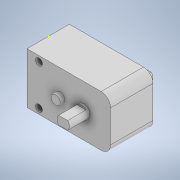
# Autodesk Inventor part: TT motor output
Saved by Autodesk Inventor 2022 (Build 260153070, 153G)
## iProperties
Created: 2021-11-27
Part Number: TT motor output
Material: Generic
Document SubType Name: Modeling
Designer: a laptop
Density: 1 g/cm^3
Appearance: Default
Author: a laptop
Autodesk Inventor part; units mm, degrees
ref_plane "YZ Plane" through (0, 0, 0) normal (1, 0, 0) x (0, 1, 0)
ref_plane "XZ Plane" through (0, 0, 0) normal (0, 1, 0) x (-1, 0, 0)
ref_plane "XY Plane" through (0, 0, 0) normal (0, 0, 1) x (1, 0, 0)
sketch "Sketch1" plane through (0, 0, 0) normal (0, 0, 1) x (1, 0, 0)
  line L0 (0, 0) -> (32.375, 0)
  line L1 (36.5, 0) -> (36.5, -4.125)
  line L2 (36.5, -22.25) -> (0, -22.25)
  line L3 (0, -22.25) -> (0, -11.125)
  line L4 (0, -11.125) -> (36.5, -11.125) construction
  line L5 (0, -11.125) -> (0, 0)
  circle A0 centre (14.5, -11.125) radius 2
  circle A1 centre (5.25, -2.375) radius 1.5
  arc A2 (36.5, -4.125) -> (32.375, 0) centre (32.375, -4.125) ccw
  line L6 (32.375, 0) -> (36.5, 0)
  line L7 (36.5, -4.125) -> (36.5, -22.25)
  arc A3 (32.375, -22.25) -> (36.5, -18.125) centre (32.375, -18.125) ccw
  circle A4 centre (5.25, -19.875) radius 1.5
  circle A5 centre (24.8, -11.125) radius 2.7
  line L8 (22.8334, -9.275) -> (26.7666, -9.275)
  line L9 (26.7666, -12.975) -> (22.8334, -12.975)
  point P0 (36.5, -18.125)
  dimension "d6" = 4
  dimension "d8" = 3
  dimension "d11" = 5.25
  dimension "d12" = 22.25
  dimension "d13" = 8.75
  dimension "d16" = 14.5
  dimension "d17" = 14
  dimension "d18" = 36.5
  dimension "d19" = 3.7
  dimension "d28" = 5.4
  dimension "d29" = 11.7
  constraints: 20 end point, 9 point on circle, 7 parallel, 6 centre point, 6 perpendicular, 6 point on line, 4 symmetric about line, 3 equal length, 3 horizontal, 2 tangent, 1 coincident, 1 horizontal alignment, 1 vertical alignment, 2 other
  measures "d6" diameter of A0
  measures "d8" diameter of A1
  measures "d11" distance from line of L5 A1.centre
  measures "d12" distance of L1.start L2.start
  measures "d13" distance from line of L4 A1.centre
  measures "d16" distance from line of L3 A0.centre
  measures "d17" distance of A3.end A2.start
  measures "d18" distance of L0.start L1.start
  measures "d19" distance between parallel lines of L9 L8
  measures "d28" diameter of A5
  measures "d29" distance from line of L7 A5.centre
extrude "Extrusion1" add sketch "Sketch1" along normal mid plane 18.5 contours L0 A2 L7 A3 L2 L3 L5
extrude "Extrusion2" add sketch "Sketch1" along normal mid plane 22.5 contours A0
extrude "Extrusion3" add sketch "Sketch1" along normal mid plane 20.5 contours A5 L9 L8 | L8 A5 | A5 L9
extrude "Extrusion4" add sketch "Sketch1" along normal mid plane 36.5 contours A5 L9 L8
sketch "Sketch2" plane through (0, -22.25, 9.25) normal (-1, 0, 0) x (0, 0, 1)
  point P0 (-9.25, 22.25)
sketch "Sketch3" plane through (0, 0, -18.25) normal (0, 0, -1) x (-1, 0, 0)
  circle A0 centre (-24.8, -11.125) radius 1
  arc A1 (-22.8334, -12.975) -> (-22.8334, -9.275) centre (-24.8, -11.125) ccw projected
  point P0 (0, 0)
  dimension "d30" = 2
  constraints: 1 centre point, 1 concentric
  measures "d30" diameter of A0
extrude "Extrusion5" cut sketch "Sketch3" against normal blind 5
body "Solid1"
